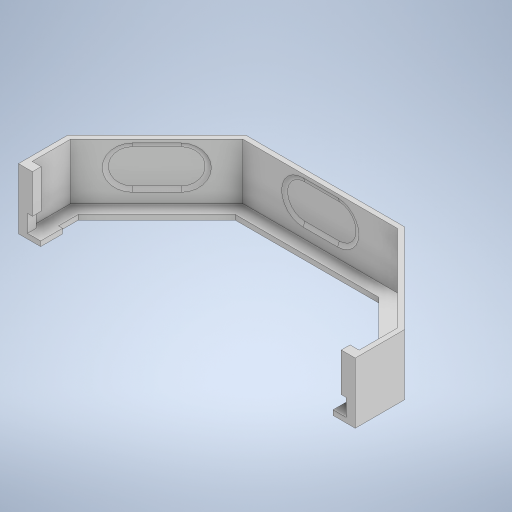
# Autodesk Inventor part: Držák TF-Luna
Saved by Autodesk Inventor 2024 (Build 280153000, 153)
## iProperties
Created: 2023-11-02
Part Number: Držák TF-Luna
Material: Všeobecné
Document SubType Name: Modeling
Designer: 42060
Density: 1 g/cm^3
Appearance: Výchozí
Author: 42060
Autodesk Inventor part; units mm, degrees
ref_plane "YZ Plane" through (0, 0, 0) normal (1, 0, 0) x (0, 1, 0)
ref_plane "XZ Plane" through (0, 0, 0) normal (0, 1, 0) x (-1, 0, 0)
ref_plane "XY Plane" through (0, 0, 0) normal (0, 0, 1) x (1, 0, 0)
ref_plane "Pracovní rovina6" through (0, 0, -9.5) normal (0, 0, -1) x (-1, 0, 0)
sketch "Náčrt19" plane through (0, 0, -9.5) normal (0, 0, -1) x (-1, 0, 0)
  circle A0 centre (20.9693, -6.1955) radius 1.75 projected
  line L0 (-19.3934, -10) -> (-23.7374, -14.344) projected
  line L1 (-13.25, -10) -> (-19.3934, -10) projected
  line L2 (-13.25, -10) -> (-13.25, -2.5) projected
  line L3 (-13.25, -2.5) -> (13.25, -2.5) projected
  line L4 (13.25, -10) -> (13.25, -2.5) projected
  line L5 (13.25, -10) -> (19.3934, -10) projected
  line L6 (19.3934, -10) -> (23.7374, -14.344) projected
  line L7 (29.0407, -9.0407) -> (23.7374, -14.344) projected
  line L8 (47.25, -27.25) -> (29.0407, -9.0407) projected
  line L9 (47.25, -36.173) -> (47.25, -27.25) projected
  line L10 (47.25, -36.173) -> (45.5, -37.923) projected
  line L11 (45.5, -37.923) -> (45.5, -47.923) projected
  line L12 (45.5, -47.923) -> (48.5, -47.923) projected
  line L13 (48.5, -37.923) -> (48.5, -47.923) projected
  line L14 (49.75, -37.923) -> (48.5, -37.923) projected
  line L15 (49.75, -26.2145) -> (49.75, -37.923) projected
  line L16 (23.5355, 0) -> (49.75, -26.2145) projected
  line L17 (-23.5355, 0) -> (23.5355, 0) projected
  line L18 (-23.5355, 0) -> (-49.75, -26.2145) projected
  line L19 (-49.75, -26.2145) -> (-49.75, -37.923) projected
  line L20 (-49.75, -37.923) -> (-48.5, -37.923) projected
  line L21 (-48.5, -37.923) -> (-48.5, -47.923) projected
  line L22 (-45.5, -47.923) -> (-48.5, -47.923) projected
  line L23 (-45.5, -37.923) -> (-45.5, -47.923) projected
  line L24 (-47.25, -36.173) -> (-45.5, -37.923) projected
  line L25 (-47.25, -36.173) -> (-47.25, -27.25) projected
  line L26 (-47.25, -27.25) -> (-29.0407, -9.0407) projected
  line L27 (-29.0407, -9.0407) -> (-23.7374, -14.344) projected
  circle A1 centre (-20.9693, -6.1955) radius 1.75 projected
  line L28 (-51.25, -25.5931) -> (-24.1569, 1.5)
  line L29 (-24.1569, 1.5) -> (24.1569, 1.5)
  line L30 (24.1569, 1.5) -> (51.25, -25.5931)
  line L31 (51.25, -25.5931) -> (51.25, -40.5931)
  line L32 (-51.25, -40.5931) -> (-51.25, -25.5931)
  line L33 (-51.25, -40.5931) -> (-48.5, -40.5931)
  line L34 (51.25, -40.5931) -> (48.5, -40.5931)
  point P0 (0, 0)
  dimension "d153" = 1.5
  dimension "d154" = 1.5
  dimension "d155" = 15
  constraints: 14 end point, 3 point on line, 1 horizontal alignment, 1 perpendicular, 3 other
  measures "d153" distance between parallel lines of L18 L28
  measures "d154" distance between parallel lines of L32 L19
  measures "d155" distance of L30.end L31.end
extrude "Vysunutí18" add sketch "Náčrt19" against normal blind 17 contours L33 L32 L28 L29 L30 L31 L34 L13 L14 L15 L16 L17 L18 L19 L20 L21
sketch "Náčrt20" plane through (0, 0, -9.5) normal (0, 0, -1) x (-1, 0, 0)
  line L0 (48.5, -37.923) -> (48.5, -40.5931) projected
  line L1 (48.5, -40.5931) -> (51.25, -40.5931) projected
  line L2 (51.25, -40.5931) -> (51.25, -25.5931) projected
  line L3 (51.25, -25.5931) -> (24.1569, 1.5) projected
  line L4 (24.1569, 1.5) -> (-24.1569, 1.5) projected
  line L5 (-24.1569, 1.5) -> (-51.25, -25.5931) projected
  line L6 (-51.25, -25.5931) -> (-51.25, -40.5931) projected
  line L7 (-51.25, -40.5931) -> (-48.5, -40.5931) projected
  line L8 (-48.5, -40.5931) -> (-48.5, -37.923) projected
  line L9 (-48.5, -37.923) -> (-49.75, -37.923) projected
  line L10 (-49.75, -37.923) -> (-49.75, -26.2145) projected
  line L11 (-49.75, -26.2145) -> (-23.5355, 0) projected
  line L12 (-23.5355, 0) -> (23.5355, 0) projected
  line L13 (23.5355, 0) -> (49.75, -26.2145) projected
  line L14 (49.75, -26.2145) -> (49.75, -37.923) projected
  line L15 (49.75, -37.923) -> (48.5, -37.923) projected
  line L16 (-45.75, -27.8713) -> (-45.75, -33.923)
  line L17 (-45.75, -33.923) -> (-44.5, -33.923)
  line L18 (-44.5, -33.923) -> (-44.5, -44.5931)
  line L19 (-44.5, -44.5931) -> (-55.25, -44.5931)
  line L20 (-55.25, -44.5931) -> (-55.25, -23.9363)
  line L21 (-55.25, -23.9363) -> (-25.8137, 5.5)
  line L22 (-25.8137, 5.5) -> (25.8137, 5.5)
  line L23 (25.8137, 5.5) -> (55.25, -23.9363)
  line L24 (55.25, -23.9363) -> (55.25, -44.5931)
  line L25 (55.25, -44.5931) -> (44.5, -44.5931)
  line L26 (44.5, -44.5931) -> (44.5, -33.923)
  line L27 (44.5, -33.923) -> (45.75, -33.923)
  line L28 (45.75, -33.923) -> (45.75, -27.8713)
  line L29 (45.75, -27.8713) -> (21.8787, -4)
  line L30 (21.8787, -4) -> (-21.8787, -4)
  line L31 (-21.8787, -4) -> (-45.75, -27.8713)
  line L32 (48.5, -40.5931) -> (44.5, -40.5931)
  line L33 (-48.5, -40.5931) -> (-44.5, -40.5931)
  point P0 (0, 0)
  dimension "d158" = 4
  constraints: 36 end point, 3 point on line, 1 perpendicular, 15 other
  measures "d158" distance between parallel lines of L10 L16
extrude "Vysunutí19" add sketch "Náčrt20" along normal blind 1.5 contours L15 L14 L13 L12 L11 L10 L9 L8 L7 L6 L5 L4 L3 L2 L1 L0 | L0 L32 L26 L27 L28 L29 L30 L31 L16 L17 L18 L33 L8 L9 L10 L11 L12 L13 L14 L15
sketch "Náčrt21" plane through (48.5, -40.5931, 7.5) normal (-1, 0, 0) x (0, 0, 1)
  line L0 (-17, 0) -> (-17, 2.6701) projected
  line L1 (-17, 0) -> (0, 0) projected
  line L2 (0, 2.6701) -> (0, 0) projected
  line L3 (-17, 2.6701) -> (0, 2.6701) projected
  line L4 (-11.75, 0) -> (-11.75, 2.6701)
  line L5 (-17, 0) -> (0, 0) projected
  point P0 (-7.5, 40.5931)
  dimension "d161" = 5.25
  constraints: 2 end point, 2 point on line, 1 perpendicular
  measures "d161" distance between parallel lines of L0 L4
extrude "Vysunutí20" add sketch "Náčrt21" along normal blind 1.5 contours L4 L3 L2 L1
sketch "Náčrt22" plane through (-48.5, -40.5931, 7.5) normal (1, 0, 0) x (0, 0, -1)
  line L0 (0, 2.6701) -> (11.75, 2.6701) projected
  line L1 (11.75, 2.6701) -> (11.75, 0) projected
  line L2 (11.75, 0) -> (0, 0) projected
  line L3 (0, 0) -> (0, 2.6701) projected
  point P0 (7.5, 40.5931)
extrude "Vysunutí21" add sketch "Náčrt22" along normal blind 1.5
sketch "Náčrt23" plane through (-23.5355, 0, 7.5) normal (0, -1, 0) x (1, 0, 0)
  line L0 (18.2855, -7.5) -> (28.7855, -7.5) construction
  line L1 (18.2855, -13) -> (28.7855, -13)
  line L2 (28.7855, -2) -> (18.2855, -2)
  arc A0 (18.2855, -2) -> (18.2855, -13) centre (18.2855, -7.5) ccw
  arc A1 (28.7855, -13) -> (28.7855, -2) centre (28.7855, -7.5) ccw
  line L3 (45.4142, -17) -> (1.6569, -17) projected
  line L4 (0, -17) -> (0, 0) projected
  line L5 (0, -8.5) -> (12.7855, -7.5) construction
  line L6 (34.2855, -7.5) -> (47.0711, -8.5) construction
  line L7 (47.0711, -17) -> (47.0711, 0) projected
  line L8 (18.2855, -1) -> (28.7855, -1)
  arc A2 (28.7855, -14) -> (28.7855, -1) centre (28.7855, -7.5) ccw
  line L9 (28.7855, -14) -> (18.2855, -14)
  arc A3 (18.2855, -1) -> (18.2855, -14) centre (18.2855, -7.5) ccw
  point P0 (23.5355, -7.5)
  point P1 (23.5355, -7.5)
  dimension "d166" = 11
  dimension "d167" = 21.5
  dimension "d168" = 4
  dimension "d169" = 1
  constraints: 16 end point, 10 point on circle, 4 centre point, 4 tangent, 3 midpoint, 2 parallel, 1 equal length, 1 horizontal, 3 other
  measures "d166" distance between parallel lines of L1 L2
  measures "d167" distance of L6.start L5.end
  measures "d168" distance between parallel lines of L3 L1
  measures "d169" distance between parallel lines of L2 L8
sketch "Náčrt24" plane through (-23.5355, 0, 7.5) normal (0.7071068, -0.7071068, 0) x (-0.7071068, -0.7071068, 0)
  line L0 (13.2864, 7.5) -> (23.7864, 7.5) construction
  line L1 (13.2864, 2) -> (23.7864, 2)
  line L2 (23.7864, 13) -> (13.2864, 13)
  arc A0 (13.2864, 13) -> (13.2864, 2) centre (13.2864, 7.5) ccw
  arc A1 (23.7864, 2) -> (23.7864, 13) centre (23.7864, 7.5) ccw
  line L3 (0, 8.5) -> (7.7864, 7.5) construction
  line L4 (29.2864, 7.5) -> (37.0729, 8.5) construction
  line L5 (13.2864, 14) -> (23.7864, 14)
  arc A2 (23.7864, 1) -> (23.7864, 14) centre (23.7864, 7.5) ccw
  line L6 (23.7864, 1) -> (13.2864, 1)
  arc A3 (13.2864, 14) -> (13.2864, 1) centre (13.2864, 7.5) ccw
  line L7 (37.0729, 17) -> (37.0729, 0) projected
  line L8 (0, 17) -> (0, 0) projected
  line L9 (0, 17) -> (37.0729, 17) projected
  point P0 (-16.6421, 7.5)
  point P1 (18.5364, 7.5)
  dimension "d170" = 11
  dimension "d171" = 21.5
  dimension "d172" = 1
  dimension "d174" = 4
  constraints: 16 end point, 10 point on circle, 4 centre point, 4 tangent, 3 midpoint, 2 parallel, 1 equal length, 1 horizontal, 3 other
  measures "d170" distance between parallel lines of L1 L2
  measures "d171" distance of L4.start L3.end
  measures "d172" distance between parallel lines of L2 L5
  measures "d174" distance between parallel lines of L9 L2
sketch "Náčrt25" plane through (49.75, -26.2145, 7.5) normal (-0.7071068, -0.7071068, 0) x (-0.7071068, 0.7071068, 0)
  line L0 (13.2864, 7.5) -> (23.7864, 7.5) construction
  line L1 (13.2864, 2) -> (23.7864, 2)
  line L2 (23.7864, 13) -> (13.2864, 13)
  arc A0 (13.2864, 13) -> (13.2864, 2) centre (13.2864, 7.5) ccw
  arc A1 (23.7864, 2) -> (23.7864, 13) centre (23.7864, 7.5) ccw
  line L3 (0, 8.5) -> (7.7864, 7.5) construction
  line L4 (29.2864, 7.5) -> (37.0729, 8.5) construction
  line L5 (13.2864, 14) -> (23.7864, 14)
  arc A2 (23.7864, 1) -> (23.7864, 14) centre (23.7864, 7.5) ccw
  line L6 (23.7864, 1) -> (13.2864, 1)
  arc A3 (13.2864, 14) -> (13.2864, 1) centre (13.2864, 7.5) ccw
  line L7 (0, 17) -> (0, 0) projected
  line L8 (37.0729, 17) -> (37.0729, 0) projected
  line L9 (1.6569, 17) -> (35.416, 17) projected
  point P0 (53.715, 7.5)
  point P1 (18.5364, 7.5)
  dimension "d175" = 11
  dimension "d176" = 21.5
  dimension "d177" = 1
  dimension "d178" = 4
  constraints: 16 end point, 10 point on circle, 4 centre point, 4 tangent, 3 midpoint, 2 parallel, 1 equal length, 1 horizontal, 3 other
  measures "d175" distance between parallel lines of L1 L2
  measures "d176" distance of L4.start L3.end
  measures "d177" distance between parallel lines of L2 L5
  measures "d178" distance between parallel lines of L9 L2
extrude "Vysunutí22" cut sketch "Náčrt23" against normal blind 0.5 contours A0 L2 A1 L1 | L8 A2 L9 A3
extrude "Vysunutí23" cut sketch "Náčrt25" against normal blind 0.5 contours A0 L2 A1 L1 | L5 A2 L6 A3
extrude "Vysunutí24" cut sketch "Náčrt24" against normal blind 0.5 contours A0 L2 A1 L1 | L5 A2 L6 A3
fillet "Zaoblení4" radius 2 12 edges at (0, 0.5, 6.5) (11.75, 0.5, 0) (0, 0.5, -6.5) (-11.75, 0.5, 0) (-36.9977, -12.7523, -6.5) (-45.3062, -21.0608, 0) (-36.9977, -12.7523, 6.5) (-28.6892, -4.4438, 0) (36.9977, -12.7523, 6.5) (45.3062, -21.0608, 0) (36.9977, -12.7523, -6.5) (28.6892, -4.4438, 0)
